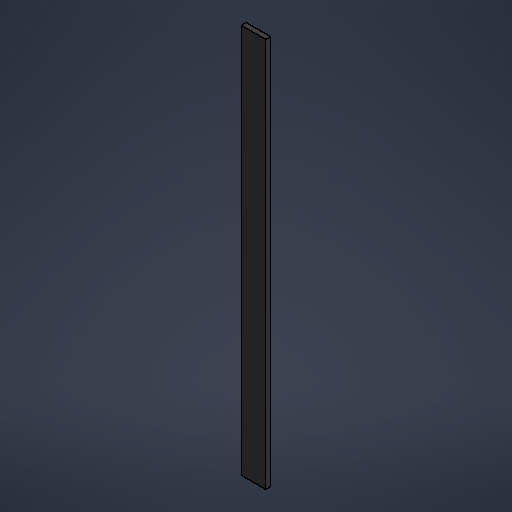
# Autodesk Inventor part: Foam Tape
Saved by Autodesk Inventor 2026 (Build 300175050, 175E)
## iProperties
Created: 2025-05-20
Part Number: Foam Tape
Material: Polyurethane Foam
Document SubType Name: Modeling
Designer: Joshua Eah
Density: 0.032 g/cm^3
Appearance: Coarse Textured - Umber
Author: Joshua Eah
Autodesk Inventor part; units mm, degrees
ref_plane "YZ Plane" through (0, 0, 0) normal (1, 0, 0) x (0, 1, 0)
ref_plane "XZ Plane" through (0, 0, 0) normal (0, 1, 0) x (-1, 0, 0)
ref_plane "XY Plane" through (0, 0, 0) normal (0, 0, 1) x (1, 0, 0)
sketch "Sketch1" plane through (0, 0, 0) normal (0, 0, 1) x (1, 0, 0)
  line L0 (0, 0) -> (5, 0)
  line L1 (5, 0) -> (5, 80)
  line L2 (5, 80) -> (0, 80)
  line L3 (0, 80) -> (0, 0)
  dimension "d0" = 5
  dimension "d1" = 80
  constraints: 8 end point, 2 parallel, 1 horizontal, 1 perpendicular
  measures "d0" distance of L2.end L1.end
  measures "d1" distance of L1.end L0.end
extrude "Extrusion1" add sketch "Sketch1" along normal blind 1
body "Solid1"
